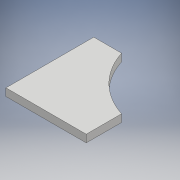
# Autodesk Inventor part: Naroznik_60x54
Saved by Autodesk Inventor 2018 (Build 220112000, 112)
## iProperties
Created: 2018-10-19
Part Number: Naroznik_60x54
Material: Ogólny
Document SubType Name: Modeling
Designer: EWA
Density: 1 g/cm^3
Appearance: Domyślna
Author: EWA
Autodesk Inventor part; units mm, degrees
ref_plane "YZ Plane" through (0, 0, 0) normal (1, 0, 0) x (0, 1, 0)
ref_plane "XZ Plane" through (0, 0, 0) normal (0, 1, 0) x (-1, 0, 0)
ref_plane "XY Plane" through (0, 0, 0) normal (0, 0, 1) x (1, 0, 0)
sketch "Szkic1" plane through (0, 0, 0) normal (0, 0, 1) x (1, 0, 0)
  line L0 (0, 0) -> (64, 0) construction
  line L1 (64, 0) -> (64, 70) construction
  line L2 (64, 70) -> (0, 70) construction
  line L3 (0, 70) -> (0, 0) construction
  line L4 (0, 0) -> (6, 0) construction
  line L5 (6, 70) -> (0, 70) construction
  line L6 (0, 70) -> (0, 0) construction
  line L7 (6, 0) -> (174, 0) construction
  line L8 (0, 0) -> (64, 0) construction
  line L9 (64, 0) -> (64, 6) construction
  line L10 (64, 6) -> (0, 6) construction
  line L11 (0, 6) -> (0, 0) construction
  line L12 (0, 6) -> (168, 6) construction
  line L13 (168, 6) -> (168, 174) construction
  line L14 (168, 174) -> (0, 174) construction
  line L15 (0, 174) -> (0, 6) construction
  line L16 (84, 174) -> (84, 6) construction
  circle A0 centre (84, 90) radius 65 construction
  line L17 (0, 0) -> (64, 0)
  line L18 (64, 0) -> (64, 28.1534)
  line L19 (0, 0) -> (0, 70)
  line L20 (0, 70) -> (22.1534, 70)
  arc A1 (22.1534, 70) -> (64, 28.1534) centre (84, 90) ccw
  dimension "d13" = 64
  dimension "d14" = 70
  dimension "d19" = 6
  dimension "d20" = 168
  dimension "d21" = 168
  dimension "d22" = 130
  constraints: 42 end point, 8 parallel, 5 horizontal, 4 point on circle, 4 point on line, 3 midpoint, 3 perpendicular, 2 centre point, 1 collinear, 1 concentric
  measures "d13" distance of L2.end L1.end
  measures "d14" distance of L1.end L0.end
  measures "d19" distance of L9.end L8.end
  measures "d20" distance of L14.end L13.end
  measures "d21" distance of L13.end L12.end
  measures "d22" diameter of A0
extrude "Wyciągnięcie proste1" add sketch "Szkic1" along normal blind 6
